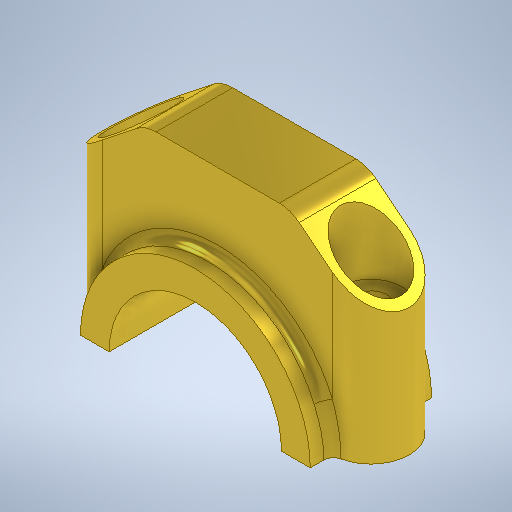
# Autodesk Inventor part: Part 4 Connecting rods cap
Saved by Autodesk Inventor 2025.2 (Build 292293000, 293)
## iProperties
Created: 2025-03-20
Part Number: Part 4 Connecting rods cap
Material: Stainless Steel
Document SubType Name: Sheet Metal
Designer: User
Density: 8 g/cm^3
Sheet Metal Rule: Default_mm
Appearance: Metal 2400F Hot
Author: User
Autodesk Inventor part; units mm, degrees
ref_plane "YZ Plane" through (0, 0, 0) normal (1, 0, 0) x (0, 1, 0)
ref_plane "XZ Plane" through (0, 0, 0) normal (0, 1, 0) x (-1, 0, 0)
ref_plane "XY Plane" through (0, 0, 0) normal (0, 0, 1) x (1, 0, 0)
sketch "Sketch1" plane through (0, 0, 0) normal (0, 0, 1) x (1, 0, 0)
  arc A0 (36, 0) -> (-36, 0) centre (0, 0) ccw
  arc A1 (27, 0) -> (-27, 0) centre (0, 0) ccw
  line L0 (-36, 0) -> (-27, 0)
  line L1 (27, 0) -> (36, 0)
  dimension "d0" = 72
  dimension "d1" = 54
  dimension "d2" = 27
  dimension "d3" = 36
  constraints: 4 end point, 4 point on circle, 2 centre point, 2 coincident, 2 horizontal
  measures "d0" diameter of A0
  measures "d1" diameter of A1
  measures "d2" radius of A1
  measures "d3" radius of A0
extrude "Extrusion1" add sketch "Sketch1" along normal mid plane 38
ref_plane "Work Plane1" through (-36, 60, 19) normal (0, -1, 0) x (1, 0, 0)
sketch "Sketch2" plane through (-36, 60, 19) normal (0, -1, 0) x (1, 0, 0)
  line L0 (9, 0) -> (63, 0) projected
  line L1 (0, -38) -> (0, 0) projected
  line L2 (0, -19) -> (72, -19) construction
  line L3 (0, -31) -> (72, -31)
  line L4 (72, -7) -> (0, -7)
  arc A0 (0, -7) -> (0, -31) centre (0, -19) ccw
  arc A1 (72, -31) -> (72, -7) centre (72, -19) ccw
  point P0 (36, -19)
  point P1 (36, -19)
  point P2 (36, 0)
  point P3 (-12, -19)
  point P4 (0, -19)
  dimension "d7" = 72
  dimension "d8" = 12
  constraints: 8 end point, 5 point on circle, 4 tangent, 3 midpoint, 2 centre point, 1 horizontal, 1 horizontal alignment, 1 parallel, 1 vertical alignment
  measures "d7" distance of L4.start L4.end
  measures "d8" radius of A1
extrude "Extrusion2" add sketch "Sketch2" along normal up to surface (60 mm away)
sketch "Sketch3" plane through (0, 0, 12) normal (0, 0, 1) x (1, 0, 0)
  arc A0 (27, 0) -> (-27, 0) centre (0, 0) ccw projected
  line L0 (-27, 0) -> (27, 0) projected
extrude "Extrusion3" cut sketch "Sketch3" against normal through all
sketch "Sketch4" plane through (0, 0, 0) normal (0, 0, 1) x (1, 0, 0)
  arc A0 (27, 0) -> (-27, 0) centre (0, 0) ccw projected
  line L0 (36, 60) -> (-36, 60) projected
  line L1 (-48, 60) -> (-48, 0) projected
  line L2 (-48, 60) -> (-48, 0) projected
  line L3 (-48, 60) -> (-36, 60) projected
  line L4 (-48, 40) -> (-22.8, 60)
  line L5 (-48, 40) -> (-48, 60)
  line L6 (0, 0) -> (0, 60) construction
  line L7 (-36, 60) -> (36, 60)
  line L8 (48, 60) -> (48, 0)
  line L9 (48, 60) -> (36, 60)
  line L10 (48, 40) -> (22.8, 60)
  dimension "d13" = 20
  dimension "d14" = 25.2
  constraints: 14 end point, 6 symmetric about line, 3 point on line, 1 collinear, 1 midpoint
  measures "d13" distance of L1.start L4.start
  measures "d14" distance of L1.start L4.end
extrude "Extrusion4" cut sketch "Sketch4" along normal through all both and the other way through all
fillet "Fillet1" radius 10 2 edges at (22.8, 60, 0) (-22.8, 60, 0)
sketch "Sketch5" plane through (-36, 0, 19) normal (0, -1, 0) x (1, 0, 0)
  arc A0 (0, -7) -> (0, -31) centre (0, -19) ccw projected
  point P0 (36, -19)
  constraints: 1 coincident
hole "Hole1" at (-36, 0, 0) direction (0, 1, 0) diameter 10 end through all
sketch "Sketch6" plane through (27, 0, -19) normal (0, -1, 0) x (1, 0, 0)
  arc A0 (9, 7) -> (9, 31) centre (9, 19) ccw projected
  point P0 (-27, 19)
  constraints: 1 coincident
hole "Hole2" at (36, 0, 0) direction (0, 1, 0) diameter 10 end through all
sketch "Sketch7" plane through (-36, 60, 19) normal (0, 1, 0) x (1, 0, 0)
  circle A0 centre (0, 19) radius 5 projected
  circle A1 centre (72, 19) radius 5 projected
  point P0 (36, 19)
  constraints: 2 coincident
hole "Hole3" at (-36, 60, 0) at (36, 60, 0) direction (0, -1, 0) diameter 10 end through all counterbore diameter 19 counterbore depth 25
fillet "Fillet2" radius 3 2 edges at (0, 36, -12) (0, 36, 12)
equation "\"d23\" = Thickness"
equation "\"BendRadius\" = Thickness"
equation "\"BendReliefWidth\" = Thickness"
equation "\"BendReliefDepth\" = 0.5 * Thickness"
equation "\"CornerReliefSize\" = 4 * Thickness"
equation "\"MinimumRemnant\" = 2 * Thickness"
equation "\"TransitionRadius\" = BendRadius"
equation "\"JacobiRadiusSize\" = BendRadius"
equation "\"GapSize\" = Thickness"
equation "\"Thickness\" = 0.5"
body "Solid1"
